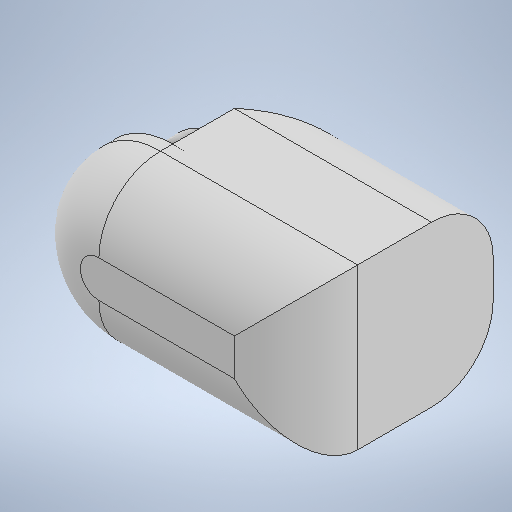
# Autodesk Inventor part: cchwytak holdeer
Saved by Autodesk Inventor 2025.2 (Build 292293000, 293)
## iProperties
Created: 2025-08-23
Part Number: cchwytak holdeer
Material: Ogólny
Document SubType Name: Modeling
Designer: IGOR
Density: 1 g/cm^3
Appearance: Domyślna
Author: IGOR
Autodesk Inventor part; units mm, degrees
ref_plane "YZ Plane" through (0, 0, 0) normal (1, 0, 0) x (0, 1, 0)
ref_plane "XZ Plane" through (0, 0, 0) normal (0, 1, 0) x (-1, 0, 0)
ref_plane "XY Plane" through (0, 0, 0) normal (0, 0, 1) x (1, 0, 0)
sketch "Szkic1" plane through (0, 0, 0) normal (0, 0, 1) x (1, 0, 0)
  circle A0 centre (0, 0) radius 10
  circle A1 centre (0, 0) radius 13
  circle A2 centre (0, 0) radius 2.45
  line L0 (0, -13) -> (32, -13)
  line L1 (32, -13) -> (32, 13)
  line L2 (32, 13) -> (0, 13)
  line L3 (-32, -13) -> (32, 13) construction
  line L4 (32, -13) -> (-32, 13) construction
  dimension "d0" = 20
  dimension "d1" = 26
  dimension "d2" = 4.9
  constraints: 10 end point, 3 centre point, 3 coincident, 2 midpoint, 2 point on circle, 1 horizontal, 1 parallel, 1 perpendicular
  measures "d0" diameter of A0
  measures "d1" diameter of A1
  measures "d2" diameter of A2
extrude "Wyciągnięcie proste1" add sketch "Szkic1" against normal blind 8 contours A0
extrude "Wyciągnięcie proste2" add sketch "Szkic1" along normal blind 12 contours A0 | A1 | A1 L2 L1 L0 | A2
extrude "Wyciągnięcie proste3" add sketch "Szkic1" against normal blind 20 contours A1 L2 L1 L0
fillet "Zaokrąglenie1" radius 10 6 edges at (16, -13, -20) (-13, 0, 12) (16, 13, 12) (16, -13, 12) (16, 13, -20) (32, 0, 12)
